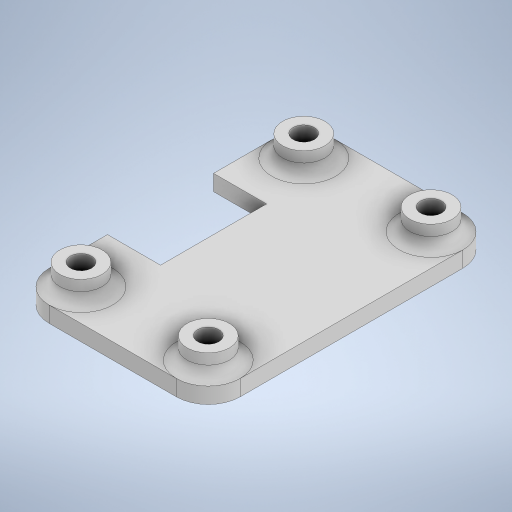
# Autodesk Inventor part: drzak_kamery2
Saved by Autodesk Inventor 2024 (Build 280153000, 153)
## iProperties
Created: 2024-05-02
Part Number: drzak_kamery2
Material: Všeobecné
Document SubType Name: Modeling
Designer: eliasla
Density: 1 g/cm^3
Appearance: Výchozí
Author: eliasla
Autodesk Inventor part; units mm, degrees
ref_plane "YZ Plane" through (0, 0, 0) normal (1, 0, 0) x (0, 1, 0)
ref_plane "XZ Plane" through (0, 0, 0) normal (0, 1, 0) x (-1, 0, 0)
ref_plane "XY Plane" through (0, 0, 0) normal (0, 0, 1) x (1, 0, 0)
sketch "Náčrt1" plane through (0, 0, 0) normal (0, 0, 1) x (1, 0, 0)
  circle A0 centre (-6, 0) radius 1
  circle A1 centre (-6, 21) radius 1
  circle A2 centre (6, 0) radius 1
  circle A3 centre (6, 21) radius 1
  arc A4 (-6, 24) -> (-9, 21) centre (-6, 21) ccw
  arc A5 (9, 21) -> (6, 24) centre (6, 21) ccw
  arc A6 (6, -3) -> (9, 0) centre (6, 0) ccw
  arc A7 (-9, 0) -> (-6, -3) centre (-6, 0) ccw
  line L0 (-6, 24) -> (6, 24)
  line L1 (9, 21) -> (9, 0)
  line L2 (-6, -3) -> (6, -3)
  line L3 (-9, 15.5) -> (-4, 15.5)
  line L4 (-9, 5.5) -> (-4, 5.5)
  line L5 (-4, 15.5) -> (-4, 5.5)
  line L6 (-9, 21) -> (-9, 15.5)
  line L7 (-9, 5.5) -> (-9, 0)
  point P0 (0, 0)
  dimension "d0" = 2
  dimension "d2" = 2
  dimension "d4" = 19
  dimension "d5" = 2
  dimension "d6" = 2
  dimension "d7" = 2
  dimension "d8" = 2
  dimension "d9" = 4.5
  dimension "d10" = 5
  constraints: 16 end point, 8 centre point, 8 point on circle, 6 tangent, 2 parallel, 1 horizontal, 1 vertical
  measures "d0" diameter of A0
  measures "d2" diameter of A1
  measures "d5" radial gap between concentric circles of A1 A4
  measures "d6" radial gap between concentric circles of A3 A5
  measures "d7" radial gap between concentric circles of A2 A6
  measures "d8" radial gap between concentric circles of A0 A7
  measures "d9" distance edge to line of A1 L3
  measures "d10" distance of L3.start L3.end
extrude "Vysunutí1" add sketch "Náčrt1" along normal blind 1.5
sketch "Náčrt3" plane through (0, 0, 1.5) normal (0, 0, 1) x (1, 0, 0)
  circle A0 centre (-6, 21) radius 1 projected
  circle A1 centre (-6, 21) radius 1
  circle A2 centre (6, 21) radius 1 projected
  circle A3 centre (6, 21) radius 1
  circle A4 centre (6, 0) radius 1 projected
  circle A5 centre (6, 0) radius 1
  circle A6 centre (-6, 0) radius 1
  circle A7 centre (-6, 21) radius 2
  circle A8 centre (6, 21) radius 2
  circle A9 centre (6, 0) radius 2
  circle A10 centre (-6, 0) radius 2
  point P0 (0, 0)
  dimension "d13" = 1
  dimension "d14" = 1
  dimension "d15" = 1
  dimension "d16" = 1
  constraints: 8 centre point, 3 coincident
  measures "d13" radial gap between concentric circles of A0 A7
  measures "d14" radial gap between concentric circles of A2 A8
  measures "d15" radial gap between concentric circles of A4 A9
  measures "d16" radial gap between concentric circles of A6 A10
extrude "Vysunutí2" add sketch "Náčrt3" along normal blind 2
fillet "Zaoblení1" radius 1 4 edges at (-8, 21, 1.5) (4, 21, 1.5) (-8, 0, 1.5) (4, 0, 1.5)
